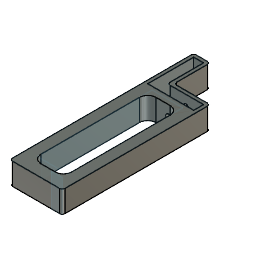
stand (Autodesk Fusion 360 design; units mm, degrees)
part number: 2025-11-26-01-15-12-232
Autodesk Fusion 360 part; units mm, degrees
sketch "Sketch1" plane through (0, 0, 0) normal (0, 0, 1) x (1, 0, 0)
  line L0 (0, 0) -> (0, 42)
  line L1 (0, 0) -> (42, 0)
  line L2 (42, 0) -> (42, 9)
  line L3 (0, 42) -> (9, 42)
  line L4 (42, 9) -> (9, 9)
  line L5 (9, 42) -> (9, 9)
  line L6 (42, 0) -> (45, 0)
  line L7 (45, 0) -> (45, 12)
  line L8 (45, 12) -> (12, 12)
  line L9 (45, 0) -> (45, -3)
  line L10 (45, -3) -> (0, -3)
  line L11 (0, -3) -> (-3, -3)
  line L12 (-3, -3) -> (-3, 45)
  line L13 (-3, 45) -> (12, 45)
  line L14 (12, 45) -> (12, 12)
  dimension "d1" = 42
  dimension "d2" = 42
  dimension "d3" = 9
  dimension "d4" = 9
  dimension "d5" = 33
  dimension "d6" = 12
  dimension "d7" = 3
  dimension "d8" = 3
  dimension "d9" = 48
  dimension "d10" = 15
  constraint coincident L0.start L1.start
  constraint vertical L0
  constraint perpendicular L0 L1
  constraint perpendicular L1 L2
  constraint perpendicular L0 L3
  constraint perpendicular L2 L4
  constraint perpendicular L2 L6
  constraint perpendicular L6 L7
  constraint perpendicular L5 L8
  constraint perpendicular L6 L9
  constraint perpendicular L9 L10
  constraint perpendicular L9 L11
  constraint perpendicular L11 L12
  constraint perpendicular L12 L13
  constraint perpendicular L8 L14
  measures "d1" distance of L0.start L0.end
  measures "d2" distance of L0.start L1.end
  measures "d3" distance of L1.end L2.end
  measures "d4" distance of L0.end L3.end
  measures "d5" distance of L2.end L4.end
  measures "d6" distance of L6.end L7.end
  measures "d7" distance of L6.end L9.end
  measures "d8" distance of L10.end L11.end
  measures "d9" distance of L11.end L12.end
  measures "d10" distance of L12.end L13.end
extrude "Extrude1" add sketch "Sketch1" along normal blind 30
sketch "Sketch2" plane through (0, -3, 0) normal (0, -1, 0) x (1, 0, 0)
  line L0 (-3, 0) -> (45, 0)
  line L1 (45, 0) -> (45, 30)
  line L2 (45, 30) -> (-3, 30)
  line L3 (-3, 30) -> (-3, 0)
  line L4 (45, 30) -> (35, 30)
  line L5 (35, 30) -> (35, 0)
  line L6 (35, 0) -> (45, 0)
  line L7 (45, 0) -> (45, 30)
  line L8 (-3, 30) -> (7, 30)
  line L9 (7, 30) -> (7, 0)
  line L10 (7, 0) -> (-3, 0)
  line L11 (-3, 0) -> (-3, 30)
  dimension "d13" = 10
  dimension "d14" = 10
  constraint horizontal L4
  constraint vertical L5
  constraint horizontal L6
  constraint vertical L7
  constraint coincident L1.end L2.start
  constraint horizontal L8
  constraint vertical L9
  constraint horizontal L10
  constraint vertical L11
  constraint coincident L2.end L3.start
  measures "d13" distance of L1.end L4.end
  measures "d14" distance of L2.end L8.end
extrude "Extrude2" add sketch "Sketch2" along normal blind 120 contours L0 L2 L3 L8 L9 L10 L11 | L0 L1 L2 L4 L5 L6 L7
sketch "Sketch3" plane through (0, -123, 0) normal (0, -1, 0) x (1, 0, 0)
  line L0 (45, 0) -> (45, 30)
  line L1 (45, 30) -> (35, 30)
  line L2 (35, 30) -> (35, 0)
  line L3 (35, 0) -> (45, 0)
sketch "Sketch4" plane through (0, -123, 0) normal (0, -1, 0) x (1, 0, 0)
  line L0 (35, 30) -> (7, 30)
  line L1 (7, 30) -> (7, 0)
  line L2 (7, 0) -> (35, 0)
  line L3 (35, 0) -> (35, 30)
  constraint horizontal L0
  constraint perpendicular L0 L1
  constraint perpendicular L1 L2
  constraint perpendicular L0 L3
extrude "Extrude3" add sketch "Sketch4" against normal blind 15
extrude "Extrude4" cut 2 faces at (16.3333, -113, 30) (1.3333, -77, 30) along direction (0, 0, -1) blind 10
sketch "Sketch5" plane through (0, 0, 20) normal (0, 0, 1) x (-1, 0, 0)
  line L0 (-7, 108) -> (-7, 3)
  line L1 (-7, 3) -> (-35, 3)
  line L2 (-35, 3) -> (-35, 108)
  line L3 (-35, 108) -> (-7, 108)
  line L4 (-42, 0) -> (0, 0)
  line L5 (0, 0) -> (0, -42)
  line L6 (0, -42) -> (-9, -42)
  line L7 (-9, -42) -> (-9, -9)
  line L8 (-9, -9) -> (-42, -9)
  line L9 (-42, -9) -> (-42, 0)
  line L10 (3, 123) -> (-45, 123)
  line L11 (-45, 123) -> (-45, -12)
  line L12 (-45, -12) -> (-12, -12)
  line L13 (-12, -12) -> (-12, -45)
  line L14 (-12, -45) -> (3, -45)
  line L15 (3, -45) -> (3, 123)
sketch "Sketch6" plane through (0, 0, 20) normal (0, 0, 1) x (-1, 0, 0)
  line L0 (-35, 108) -> (-35, 112)
  line L1 (-35, 112) -> (-7, 112)
  line L2 (-7, 112) -> (-7, 108)
  line L3 (-7, 108) -> (-35, 108)
  constraint vertical L0
  constraint perpendicular L0 L1
  constraint perpendicular L1 L2
  constraint perpendicular L0 L3
extrude "Extrude5" cut sketch "Sketch6" against normal blind 20
sketch "Sketch7" plane through (0, 0, 20) normal (0, 0, 1) x (-1, 0, 0)
  line L0 (-7, 3) -> (-35, 3)
  line L1 (-35, 3) -> (-35, 7)
  line L2 (-35, 7) -> (-7, 7)
  line L3 (-7, 7) -> (-7, 3)
  constraint horizontal L0
  constraint vertical L1
  constraint horizontal L2
  constraint vertical L3
extrude "Extrude6" add sketch "Sketch7" against normal blind 20
fillet "Fillet1" radius 2.5 1 edges at (12, 45, 10)
fillet "Fillet2" radius 2.5 1 edges at (-3, 45, 10)
fillet "Fillet3" radius 2.5 1 edges at (45, 12, 10)
fillet "Fillet4" radius 2.5 1 edges at (12, 12, 10)
fillet "Fillet5" radius 2.5 1 edges at (45, -123, 10)
fillet "Fillet6" radius 2.5 1 edges at (-3, -123, 10)
fillet "Fillet7" radius 2.5 1 edges at (9, 9, 10)
fillet "Fillet8" radius 7.5 2 edges at (35, -112, 10) (7, -112, 10)
fillet "Fillet9" radius 7.5 2 edges at (7, -7, 10) (35, -7, 10)
sketch "Sketch8" plane through (0, 0, 0) normal (1, 0, 0) x (0, 1, 0)
sketch "Sketch9" plane through (0, 0, 20) normal (0, 0, 1) x (-1, 0, 0)
sketch "Sketch10" plane through (7, 0, 0) normal (1, 0, 0) x (0, 1, 0)
  line L0 (-14.5, 0) -> (-14.5, 20)
  line L1 (-14.5, 20) -> (-104.5, 20)
  line L2 (-104.5, 20) -> (-104.5, 0)
  line L3 (-104.5, 0) -> (-14.5, 0)
sketch "Sketch11" plane through (0, 0, 20) normal (0, 0, 1) x (-1, 0, 0)
sketch "Sketch12" plane through (0, 12, 0) normal (0, 1, 0) x (-1, 0, 0)
  line L0 (-14.5, 0) -> (-14.5, 20)
  line L1 (-14.5, 20) -> (-42.5, 20)
  line L2 (-42.5, 20) -> (-42.5, 0)
  line L3 (-42.5, 0) -> (-14.5, 0)
  line L4 (-45, 10) -> (-26, 10)
  circle A0 centre (-26, 10) radius 2.5
  dimension "d43" = 5
  constraint perpendicular L2 L4
  constraint coincident L4.end A0.centre
  measures "d43" diameter of A0
extrude "Extrude7" cut sketch "Sketch12" against normal blind 28 contours A0
